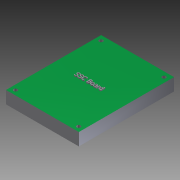
# Autodesk Inventor part: ssc board
Saved by Autodesk Inventor 2012 (Build 160160000, 160)
## iProperties
Created: 2013-12-07
Part Number: ssc board
Material: Default
Document SubType Name: Modeling
Designer: Irwan Haryanto
Density: 1 g/cm^3
Author: Irwan Haryanto
Autodesk Inventor part; units mm, degrees
ref_plane "YZ Plane" through (0, 0, 0) normal (1, 0, 0) x (0, 1, 0)
ref_plane "XZ Plane" through (0, 0, 0) normal (0, 1, 0) x (-1, 0, 0)
ref_plane "XY Plane" through (0, 0, 0) normal (0, 0, 1) x (1, 0, 0)
sketch "Sketch1" plane through (0, 0, 0) normal (0, 0, 1) x (1, 0, 0)
  line L0 (-29.3713, 37.636) -> (29.0687, 37.636)
  line L1 (29.0687, 37.636) -> (29.0687, -38.664)
  line L2 (29.0687, -38.664) -> (-29.3713, -38.664)
  line L3 (-29.3713, -38.664) -> (-29.3713, 37.636)
  circle A0 centre (25.0687, 33.636) radius 1.5
  circle A1 centre (-25.4813, 33.636) radius 1.5
  circle A2 centre (25.0687, -34.864) radius 1.5
  circle A3 centre (-25.4813, -34.864) radius 1.5
  line L4 (-12.1842, 1.9609) -> (9.9418, 1.9609) construction
  line L5 (9.9418, 1.9609) -> (9.9418, 9.0457) construction
  line L6 (9.9418, 9.0457) -> (-12.1842, 9.0457) construction
  line L7 (-12.1842, 9.0457) -> (-12.1842, 1.9609) construction
  point P0 (0, 0)
  point P1 (-8.4313, -38.664)
  point P2 (11.5687, -38.664)
  point P3 (0, 0)
  dimension "d0" = 3
  dimension "d1" = 3
  dimension "d2" = 3
  dimension "d3" = 58.44
  dimension "d4" = 76.3
  dimension "d5" = 50.55
  dimension "d6" = 68.5
  dimension "d7" = 68.5
  dimension "d8" = 50.55
  constraints: 8 end point, 4 centre point, 2 parallel, 2 point on line, 1 horizontal, 1 perpendicular, 2 other
  measures "d0" diameter of A1
  measures "d1" diameter of A2
  measures "d2" diameter of A3
  measures "d3" distance of L0.start L0.end
  measures "d4" distance of L0.end L1.end
  measures "d5" distance of A0.centre A1.centre
  measures "d6" distance of A2.centre A0.centre
  measures "d7" distance of A3.centre A1.centre
  measures "d8" distance of A2.centre A3.centre
extrude "Extrusion1" add sketch "Sketch1" along normal blind 10 contours L0 L1 L2 L3 | A0 | A1 | A2 | A3
sketch "Sketch2" plane through (0, 0, 10) normal (0, 0, 1) x (1, 0, 0)
  line L0 (-29.3713, 37.636) -> (29.0687, 37.636)
  line L1 (29.0687, 37.636) -> (29.0687, -38.664)
  line L2 (29.0687, -38.664) -> (-29.3713, -38.664)
  line L3 (-29.3713, -38.664) -> (-29.3713, 37.636)
  circle A0 centre (25.0687, 33.636) radius 1.5
  circle A1 centre (-25.4813, 33.636) radius 1.5
  circle A2 centre (25.0687, -34.864) radius 1.5
  circle A3 centre (-25.4813, -34.864) radius 1.5
  line L4 (-12.1842, 1.9609) -> (9.9418, 1.9609) construction
  line L5 (9.9418, 1.9609) -> (9.9418, 9.0457) construction
  line L6 (9.9418, 9.0457) -> (-12.1842, 9.0457) construction
  line L7 (-12.1842, 9.0457) -> (-12.1842, 1.9609) construction
  spline S0 degree 2 poles (-10.854, -1.7575) (-11.2341, -1.7575) (-11.7673, -1.5986) (-12.0027, -1.4852) knots 0 0 0 1 2 2 2
  line L8 (-12.0027, -1.4852) -> (-12.0027, -0.9009)
  line L9 (-12.0027, -0.9009) -> (-11.9687, -0.9009)
  spline S1 degree 2 poles (-11.9687, -0.9009) (-11.7389, -1.1165) (-11.1575, -1.3547) (-10.888, -1.3547) knots 0 0 0 1 2 2 2
  spline S2 degree 2 poles (-10.888, -1.3547) (-10.5023, -1.3547) (-10.1081, -1.0342) (-10.1081, -0.7704) knots 0 0 0 1 2 2 2
  spline S3 degree 2 poles (-10.1081, -0.7704) (-10.1081, -0.5605) (-10.3151, -0.2996) (-10.5392, -0.2344) knots 0 0 0 1 2 2 2
  spline S4 degree 2 poles (-10.5392, -0.2344) (-10.7008, -0.189) (-10.9703, -0.1266) (-11.1717, -0.0755) knots 0 0 0 1 2 2 2
  spline S5 degree 2 poles (-11.1717, -0.0755) (-11.3532, -0.0273) (-11.6397, 0.1173) (-11.7503, 0.2336) knots 0 0 0 1 2 2 2
  spline S6 degree 2 poles (-11.7503, 0.2336) (-11.8581, 0.3499) (-11.9772, 0.6619) (-11.9772, 0.8661) knots 0 0 0 1 2 2 2
  spline S7 degree 2 poles (-11.9772, 0.8661) (-11.9772, 1.2916) (-11.3135, 1.8673) (-10.8001, 1.8673) knots 0 0 0 1 2 2 2
  spline S8 degree 2 poles (-10.8001, 1.8673) (-10.5051, 1.8673) (-9.9833, 1.751) (-9.7592, 1.6404) knots 0 0 0 1 2 2 2
  line L10 (-9.7592, 1.6404) -> (-9.7592, 1.0845)
  line L11 (-9.7592, 1.0845) -> (-9.7932, 1.0845)
  spline S9 degree 2 poles (-9.7932, 1.0845) (-9.9606, 1.2377) (-10.4825, 1.4646) (-10.7689, 1.4646) knots 0 0 0 1 2 2 2
  spline S10 degree 2 poles (-10.7689, 1.4646) (-11.0923, 1.4646) (-11.4922, 1.1611) (-11.4922, 0.9143) knots 0 0 0 1 2 2 2
  spline S11 degree 2 poles (-11.4922, 0.9143) (-11.4922, 0.6931) (-11.2568, 0.4293) (-11.0355, 0.3698) knots 0 0 0 1 2 2 2
  spline S12 degree 2 poles (-11.0355, 0.3698) (-10.888, 0.3301) (-10.4598, 0.228) (-10.3179, 0.1854) knots 0 0 0 1 2 2 2
  spline S13 degree 2 poles (-10.3179, 0.1854) (-9.9577, 0.0748) (-9.6231, -0.3705) (-9.6231, -0.6967) knots 0 0 0 1 2 2 2
  spline S14 degree 2 poles (-9.6231, -0.6967) (-9.6231, -0.9037) (-9.7904, -1.3008) (-9.9407, -1.4398) knots 0 0 0 1 2 2 2
  spline S15 degree 2 poles (-9.9407, -1.4398) (-10.1081, -1.593) (-10.5335, -1.7575) (-10.854, -1.7575) knots 0 0 0 1 2 2 2
  spline S16 degree 2 poles (-8.1737, -1.7575) (-8.5538, -1.7575) (-9.087, -1.5986) (-9.3224, -1.4852) knots 0 0 0 1 2 2 2
  line L12 (-9.3224, -1.4852) -> (-9.3224, -0.9009)
  line L13 (-9.3224, -0.9009) -> (-9.2884, -0.9009)
  spline S17 degree 2 poles (-9.2884, -0.9009) (-9.0586, -1.1165) (-8.4772, -1.3547) (-8.2077, -1.3547) knots 0 0 0 1 2 2 2
  spline S18 degree 2 poles (-8.2077, -1.3547) (-7.822, -1.3547) (-7.4278, -1.0342) (-7.4278, -0.7704) knots 0 0 0 1 2 2 2
  spline S19 degree 2 poles (-7.4278, -0.7704) (-7.4278, -0.5605) (-7.6348, -0.2996) (-7.8589, -0.2344) knots 0 0 0 1 2 2 2
  spline S20 degree 2 poles (-7.8589, -0.2344) (-8.0205, -0.189) (-8.29, -0.1266) (-8.4914, -0.0755) knots 0 0 0 1 2 2 2
  spline S21 degree 2 poles (-8.4914, -0.0755) (-8.6729, -0.0273) (-8.9594, 0.1173) (-9.07, 0.2336) knots 0 0 0 1 2 2 2
  spline S22 degree 2 poles (-9.07, 0.2336) (-9.1778, 0.3499) (-9.2969, 0.6619) (-9.2969, 0.8661) knots 0 0 0 1 2 2 2
  spline S23 degree 2 poles (-9.2969, 0.8661) (-9.2969, 1.2916) (-8.6332, 1.8673) (-8.1198, 1.8673) knots 0 0 0 1 2 2 2
  spline S24 degree 2 poles (-8.1198, 1.8673) (-7.8248, 1.8673) (-7.303, 1.751) (-7.0789, 1.6404) knots 0 0 0 1 2 2 2
  line L14 (-7.0789, 1.6404) -> (-7.0789, 1.0845)
  line L15 (-7.0789, 1.0845) -> (-7.1129, 1.0845)
  spline S25 degree 2 poles (-7.1129, 1.0845) (-7.2803, 1.2377) (-7.8021, 1.4646) (-8.0886, 1.4646) knots 0 0 0 1 2 2 2
  spline S26 degree 2 poles (-8.0886, 1.4646) (-8.412, 1.4646) (-8.8119, 1.1611) (-8.8119, 0.9143) knots 0 0 0 1 2 2 2
  spline S27 degree 2 poles (-8.8119, 0.9143) (-8.8119, 0.6931) (-8.5765, 0.4293) (-8.3552, 0.3698) knots 0 0 0 1 2 2 2
  spline S28 degree 2 poles (-8.3552, 0.3698) (-8.2077, 0.3301) (-7.7795, 0.228) (-7.6376, 0.1854) knots 0 0 0 1 2 2 2
  spline S29 degree 2 poles (-7.6376, 0.1854) (-7.2774, 0.0748) (-6.9427, -0.3705) (-6.9427, -0.6967) knots 0 0 0 1 2 2 2
  spline S30 degree 2 poles (-6.9427, -0.6967) (-6.9427, -0.9037) (-7.1101, -1.3008) (-7.2604, -1.4398) knots 0 0 0 1 2 2 2
  spline S31 degree 2 poles (-7.2604, -1.4398) (-7.4278, -1.593) (-7.8532, -1.7575) (-8.1737, -1.7575) knots 0 0 0 1 2 2 2
  spline S32 degree 2 poles (-5.102, -1.7575) (-5.4423, -1.7575) (-6.0181, -1.5277) (-6.228, -1.298) knots 0 0 0 1 2 2 2
  spline S33 degree 2 poles (-6.228, -1.298) (-6.4379, -1.0711) (-6.6676, -0.3904) (-6.6676, 0.0521) knots 0 0 0 1 2 2 2
  spline S34 degree 2 poles (-6.6676, 0.0521) (-6.6676, 0.4917) (-6.4436, 1.1441) (-6.2308, 1.3852) knots 0 0 0 1 2 2 2
  spline S35 degree 2 poles (-6.2308, 1.3852) (-6.0209, 1.6206) (-5.448, 1.8673) (-5.0935, 1.8673) knots 0 0 0 1 2 2 2
  spline S36 degree 2 poles (-5.0935, 1.8673) (-4.9176, 1.8673) (-4.6085, 1.8163) (-4.478, 1.7766) knots 0 0 0 1 2 2 2
  spline S37 degree 2 poles (-4.478, 1.7766) (-4.3645, 1.7397) (-4.1291, 1.6348) (-4.0128, 1.5724) knots 0 0 0 1 2 2 2
  line L16 (-4.0128, 1.5724) -> (-4.0128, 1.0108)
  line L17 (-4.0128, 1.0108) -> (-4.0497, 1.0108)
  spline S38 degree 2 poles (-4.0497, 1.0108) (-4.1121, 1.0675) (-4.305, 1.2263) (-4.444, 1.3029) knots 0 0 0 1 2 2 2
  spline S39 degree 2 poles (-4.444, 1.3029) (-4.5773, 1.3767) (-4.8921, 1.4703) (-5.0963, 1.4703) knots 0 0 0 1 2 2 2
  spline S40 degree 2 poles (-5.0963, 1.4703) (-5.3204, 1.4703) (-5.7203, 1.2859) (-5.8706, 1.11) knots 0 0 0 1 2 2 2
  spline S41 degree 2 poles (-5.8706, 1.11) (-6.0181, 0.9314) (-6.1826, 0.3896) (-6.1826, 0.0521) knots 0 0 0 1 2 2 2
  spline S42 degree 2 poles (-6.1826, 0.0521) (-6.1826, -0.3081) (-6.0096, -0.8272) (-5.8593, -1.0058) knots 0 0 0 1 2 2 2
  spline S43 degree 2 poles (-5.8593, -1.0058) (-5.7118, -1.1789) (-5.3175, -1.3547) (-5.0963, -1.3547) knots 0 0 0 1 2 2 2
  spline S44 degree 2 poles (-5.0963, -1.3547) (-4.8949, -1.3547) (-4.5517, -1.2554) (-4.4184, -1.1817) knots 0 0 0 1 2 2 2
  spline S45 degree 2 poles (-4.4184, -1.1817) (-4.2908, -1.1079) (-4.1008, -0.9548) (-4.0469, -0.9009) knots 0 0 0 1 2 2 2
  line L18 (-4.0469, -0.9009) -> (-4.0128, -0.9009)
  line L19 (-4.0128, -0.9009) -> (-4.0128, -1.4568)
  spline S46 degree 2 poles (-4.0128, -1.4568) (-4.1291, -1.5107) (-4.3333, -1.61) (-4.478, -1.6554) knots 0 0 0 1 2 2 2
  spline S47 degree 2 poles (-4.478, -1.6554) (-4.6312, -1.7064) (-4.8921, -1.7575) (-5.102, -1.7575) knots 0 0 0 1 2 2 2
  spline S48 degree 2 poles (0.2983, -0.6201) (0.2983, -0.881) (0.0998, -1.281) (-0.0647, -1.4114) knots 0 0 0 1 2 2 2
  spline S49 degree 2 poles (-0.0647, -1.4114) (-0.2632, -1.5646) (-0.7142, -1.6951) (-1.0716, -1.6951) knots 0 0 0 1 2 2 2
  line L20 (-1.0716, -1.6951) -> (-2.0756, -1.6951)
  line L21 (-2.0756, -1.6951) -> (-2.0756, 1.8049)
  line L22 (-2.0756, 1.8049) -> (-1.1482, 1.8049)
  spline S50 degree 2 poles (-1.1482, 1.8049) (-0.7738, 1.8049) (-0.3994, 1.7567) (-0.2292, 1.6631) knots 0 0 0 1 2 2 2
  spline S51 degree 2 poles (-0.2292, 1.6631) (-0.0392, 1.5639) (0.1338, 1.2377) (0.1338, 1.0164) knots 0 0 0 1 2 2 2
  spline S52 degree 2 poles (0.1338, 1.0164) (0.1338, 0.7697) (-0.1271, 0.3783) (-0.3568, 0.2677) knots 0 0 0 1 2 2 2
  line L23 (-0.3568, 0.2677) -> (-0.3568, 0.2506)
  spline S53 degree 2 poles (-0.3568, 0.2506) (-0.0449, 0.1656) (0.2983, -0.2854) (0.2983, -0.6201) knots 0 0 0 1 2 2 2
  spline S54 degree 2 poles (-0.1867, -0.64) (-0.1867, -0.4414) (-0.3001, -0.1861) (-0.4703, -0.0954) knots 0 0 0 1 2 2 2
  spline S55 degree 2 poles (-0.4703, -0.0954) (-0.5809, -0.0387) (-0.8419, -0.0046) (-1.0829, -0.0046) knots 0 0 0 1 2 2 2
  line L24 (-1.0829, -0.0046) -> (-1.6105, -0.0046)
  line L25 (-1.6105, -0.0046) -> (-1.6105, -1.298)
  line L26 (-1.6105, -1.298) -> (-1.2333, -1.298)
  spline S56 degree 2 poles (-1.2333, -1.298) (-0.9269, -1.298) (-0.5752, -1.2413) (-0.4391, -1.1505) knots 0 0 0 1 2 2 2
  spline S57 degree 2 poles (-0.4391, -1.1505) (-0.3086, -1.0569) (-0.1867, -0.8243) (-0.1867, -0.64) knots 0 0 0 1 2 2 2
  spline S58 degree 2 poles (-0.3512, 0.9512) (-0.3512, 1.076) (-0.4363, 1.2632) (-0.5299, 1.3171) knots 0 0 0 1 2 2 2
  spline S59 degree 2 poles (-0.5299, 1.3171) (-0.6433, 1.3795) (-0.9184, 1.4079) (-1.1652, 1.4079) knots 0 0 0 1 2 2 2
  line L27 (-1.1652, 1.4079) -> (-1.6105, 1.4079)
  line L28 (-1.6105, 1.4079) -> (-1.6105, 0.3839)
  line L29 (-1.6105, 0.3839) -> (-1.0829, 0.3839)
  spline S60 degree 2 poles (-1.0829, 0.3839) (-0.8645, 0.3839) (-0.6575, 0.4293) (-0.5469, 0.5002) knots 0 0 0 1 2 2 2
  spline S61 degree 2 poles (-0.5469, 0.5002) (-0.4391, 0.5683) (-0.3512, 0.7867) (-0.3512, 0.9512) knots 0 0 0 1 2 2 2
  spline S62 degree 2 poles (2.8851, -0.3819) (2.8851, -1.0455) (2.2469, -1.7688) (1.7137, -1.7688) knots 0 0 0 1 2 2 2
  spline S63 degree 2 poles (1.7137, -1.7688) (1.1663, -1.7688) (0.5394, -1.0229) (0.5394, -0.3819) knots 0 0 0 1 2 2 2
  spline S64 degree 2 poles (0.5394, -0.3819) (0.5394, 0.2762) (1.1861, 1.0051) (1.7137, 1.0051) knots 0 0 0 1 2 2 2
  spline S65 degree 2 poles (1.7137, 1.0051) (2.2469, 1.0051) (2.8851, 0.279) (2.8851, -0.3819) knots 0 0 0 1 2 2 2
  spline S66 degree 2 poles (2.4284, -0.3819) (2.4284, 0.1287) (2.0568, 0.625) (1.7137, 0.625) knots 0 0 0 1 2 2 2
  spline S67 degree 2 poles (1.7137, 0.625) (1.3705, 0.625) (0.9961, 0.1287) (0.9961, -0.3819) knots 0 0 0 1 2 2 2
  spline S68 degree 2 poles (0.9961, -0.3819) (0.9961, -0.8782) (1.3705, -1.3887) (1.7137, -1.3887) knots 0 0 0 1 2 2 2
  spline S69 degree 2 poles (1.7137, -1.3887) (2.054, -1.3887) (2.4284, -0.8867) (2.4284, -0.3819) knots 0 0 0 1 2 2 2
  spline S70 degree 2 poles (4.8024, -1.4171) (4.7485, -1.4568) (4.567, -1.5986) (4.4819, -1.6412) knots 0 0 0 1 2 2 2
  spline S71 degree 2 poles (4.4819, -1.6412) (4.3656, -1.7036) (4.1472, -1.7688) (3.9487, -1.7688) knots 0 0 0 1 2 2 2
  spline S72 degree 2 poles (3.9487, -1.7688) (3.787, -1.7688) (3.4949, -1.6468) (3.3842, -1.5362) knots 0 0 0 1 2 2 2
  spline S73 degree 2 poles (3.3842, -1.5362) (3.2793, -1.4284) (3.1517, -1.1108) (3.1517, -0.9349) knots 0 0 0 1 2 2 2
  spline S74 degree 2 poles (3.1517, -0.9349) (3.1517, -0.6626) (3.3814, -0.2769) (3.631, -0.1663) knots 0 0 0 1 2 2 2
  spline S75 degree 2 poles (3.631, -0.1663) (3.8522, -0.0642) (4.4535, 0.0124) (4.8024, 0.0322) knots 0 0 0 1 2 2 2
  line L30 (4.8024, 0.0322) -> (4.8024, 0.1173)
  spline S76 degree 2 poles (4.8024, 0.1173) (4.8024, 0.2705) (4.7088, 0.4605) (4.6237, 0.5144) knots 0 0 0 1 2 2 2
  spline S77 degree 2 poles (4.6237, 0.5144) (4.5386, 0.5683) (4.2947, 0.6023) (4.1642, 0.6023) knots 0 0 0 1 2 2 2
  spline S78 degree 2 poles (4.1642, 0.6023) (4.0111, 0.6023) (3.597, 0.5116) (3.3899, 0.4237) knots 0 0 0 1 2 2 2
  line L31 (3.3899, 0.4237) -> (3.3644, 0.4237)
  line L32 (3.3644, 0.4237) -> (3.3644, 0.8746)
  spline S79 degree 2 poles (3.3644, 0.8746) (3.4863, 0.9087) (3.943, 0.9938) (4.1671, 0.9938) knots 0 0 0 1 2 2 2
  spline S80 degree 2 poles (4.1671, 0.9938) (4.4393, 0.9938) (4.8109, 0.9087) (4.9584, 0.7981) knots 0 0 0 1 2 2 2
  spline S81 degree 2 poles (4.9584, 0.7981) (5.103, 0.6903) (5.2449, 0.3471) (5.2449, 0.1003) knots 0 0 0 1 2 2 2
  line L33 (5.2449, 0.1003) -> (5.2449, -1.6951)
  line L34 (5.2449, -1.6951) -> (4.8024, -1.6951)
  line L35 (4.8024, -1.6951) -> (4.8024, -1.4171)
  line L36 (4.8024, -1.0484) -> (4.8024, -0.3195)
  spline S82 degree 2 poles (4.8024, -0.3195) (4.6436, -0.3336) (4.1642, -0.3819) (4.0139, -0.4272) knots 0 0 0 1 2 2 2
  spline S83 degree 2 poles (4.0139, -0.4272) (3.838, -0.4811) (3.6083, -0.7052) (3.6083, -0.9037) knots 0 0 0 1 2 2 2
  spline S84 degree 2 poles (3.6083, -0.9037) (3.6083, -1.1306) (3.8636, -1.3604) (4.1075, -1.3604) knots 0 0 0 1 2 2 2
  spline S85 degree 2 poles (4.1075, -1.3604) (4.3145, -1.3604) (4.6549, -1.1817) (4.8024, -1.0484) knots 0 0 0 1 2 2 2
  line L37 (7.2586, 0.4577) -> (7.2359, 0.4577)
  spline S86 degree 2 poles (7.2359, 0.4577) (7.1849, 0.4719) (7.0743, 0.4775) (6.9977, 0.4775) knots 0 0 0 1 2 2 2
  spline S87 degree 2 poles (6.9977, 0.4775) (6.819, 0.4775) (6.4673, 0.3216) (6.3085, 0.1684) knots 0 0 0 1 2 2 2
  line L38 (6.3085, 0.1684) -> (6.3085, -1.6951)
  line L39 (6.3085, -1.6951) -> (5.866, -1.6951)
  line L40 (5.866, -1.6951) -> (5.866, 0.9314)
  line L41 (5.866, 0.9314) -> (6.3085, 0.9314)
  line L42 (6.3085, 0.9314) -> (6.3085, 0.5399)
  spline S88 degree 2 poles (6.3085, 0.5399) (6.5496, 0.7555) (6.9098, 0.9314) (7.0799, 0.9314) knots 0 0 0 1 2 2 2
  spline S89 degree 2 poles (7.0799, 0.9314) (7.148, 0.9314) (7.2161, 0.9257) (7.2586, 0.9172) knots 0 0 0 1 2 2 2
  line L43 (7.2586, 0.9172) -> (7.2586, 0.4577)
  line L44 (9.6213, -1.6951) -> (9.1788, -1.6951)
  line L45 (9.1788, -1.6951) -> (9.1788, -1.4284)
  spline S90 degree 2 poles (9.1788, -1.4284) (9.0767, -1.5135) (8.9264, -1.627) (8.8243, -1.6752) knots 0 0 0 1 2 2 2
  spline S91 degree 2 poles (8.8243, -1.6752) (8.7307, -1.7206) (8.5293, -1.7688) (8.396, -1.7688) knots 0 0 0 1 2 2 2
  spline S92 degree 2 poles (8.396, -1.7688) (8.1804, -1.7688) (7.8174, -1.5901) (7.6898, -1.4171) knots 0 0 0 1 2 2 2
  spline S93 degree 2 poles (7.6898, -1.4171) (7.5621, -1.2441) (7.4203, -0.7336) (7.4203, -0.4017) knots 0 0 0 1 2 2 2
  spline S94 degree 2 poles (7.4203, -0.4017) (7.4203, -0.0557) (7.599, 0.4492) (7.755, 0.6392) knots 0 0 0 1 2 2 2
  spline S95 degree 2 poles (7.755, 0.6392) (7.8996, 0.8094) (8.3052, 1.0051) (8.5293, 1.0051) knots 0 0 0 1 2 2 2
  spline S96 degree 2 poles (8.5293, 1.0051) (8.725, 1.0051) (9.0171, 0.9172) (9.1788, 0.8264) knots 0 0 0 1 2 2 2
  line L46 (9.1788, 0.8264) -> (9.1788, 1.9609)
  line L47 (9.1788, 1.9609) -> (9.6213, 1.9609)
  line L48 (9.6213, 1.9609) -> (9.6213, -1.6951)
  line L49 (9.1788, -1.0569) -> (9.1788, 0.4605)
  spline S97 degree 2 poles (9.1788, 0.4605) (9.0143, 0.5399) (8.7534, 0.5995) (8.603, 0.5995) knots 0 0 0 1 2 2 2
  spline S98 degree 2 poles (8.603, 0.5995) (8.2627, 0.5995) (7.8769, 0.089) (7.8769, -0.3932) knots 0 0 0 1 2 2 2
  spline S99 degree 2 poles (7.8769, -0.3932) (7.8769, -0.8584) (8.1719, -1.349) (8.4981, -1.349) knots 0 0 0 1 2 2 2
  spline S100 degree 2 poles (8.4981, -1.349) (8.6711, -1.349) (9.0228, -1.1902) (9.1788, -1.0569) knots 0 0 0 1 2 2 2
  point P0 (0, 0)
  point P1 (-8.4313, -38.664)
  point P2 (11.5687, -38.664)
  point P3 (0, 0)
  dimension "d11" = 3
  dimension "d12" = 3
  dimension "d13" = 3
  dimension "d14" = 58.44
  dimension "d15" = 76.3
  dimension "d16" = 50.55
  dimension "d17" = 68.5
  dimension "d18" = 68.5
  dimension "d19" = 50.55
  constraints: 8 end point, 4 centre point, 2 parallel, 2 point on line, 1 horizontal, 1 perpendicular, 2 other
  measures "d11" diameter of A1
  measures "d12" diameter of A2
  measures "d13" diameter of A3
  measures "d14" distance of L0.start L0.end
  measures "d15" distance of L0.end L1.end
  measures "d16" distance of A0.centre A1.centre
  measures "d17" distance of A2.centre A0.centre
  measures "d18" distance of A3.centre A1.centre
  measures "d19" distance of A2.centre A3.centre
hole "Hole1" at (-25.4813, 33.636, 10) at (25.0687, 33.636, 10) at (25.0687, -34.864, 10) at (-25.4813, -34.864, 10) direction (0, 0, -1) diameter 3 end through all
emboss "Emboss1" sketch "Sketch2" operation add depth 1 direction (0, 0, -1) contours S0 L8 L9 S1 S2 S3 S4 S5 S6 S7 S8 L10 L11 S9 S10 S11 S12 S13 S14 S15 | S16 L12 L13 S17 S18 S19 S20 S21 S22 S23 S24 L14 L15 S25 S26 S27 S28 S29 S30 S31 | S32 S33 S34 S35 S36 S37 L16 L17 S38 S39 S40 S41 S42 S43 S44 S45 L18 L19 S46 S47 | S48 S49 L20 L21 L22 S50 S51 S52 L23 S53 | S62 S63 S64 S65 | S70 S71 S72 S73 S74 S75 L30 S76 S77 S78 L31 L32 S79 S80 S81 L33 L34 L35 | L37 S86 S87 L38 L39 L40 L41 L42 S88 S89 L43 | L44 L45 S90 S91 S92 S93 S94 S95 S96 L46 L47 L48
body "Solid1"
